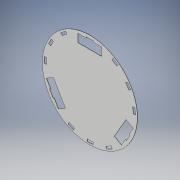
# Autodesk Inventor part: Part2
Saved by Autodesk Inventor 2019 (Build 230136000, 136)
## iProperties
Created: 2021-01-08
Part Number: Part2
Material: Generic
Document SubType Name: Modeling
Designer: DELL
Density: 1 g/cm^3
Appearance: Default
Author: DELL
Autodesk Inventor part; units mm, degrees
ref_plane "YZ Plane" through (0, 0, 0) normal (1, 0, 0) x (0, 1, 0)
ref_plane "XZ Plane" through (0, 0, 0) normal (0, 1, 0) x (-1, 0, 0)
ref_plane "XY Plane" through (0, 0, 0) normal (0, 0, 1) x (1, 0, 0)
sketch "Sketch1" plane through (0, 0, 0) normal (0, 0, 1) x (1, 0, 0)
  circle A0 centre (0, 0) radius 200
  line L0 (0, 187.7709) -> (15, 187.7709)
  line L1 (15, 187.7709) -> (15, 182.7709)
  line L2 (15, 182.7709) -> (50, 182.7709)
  line L3 (50, 182.7709) -> (50, 147.7709)
  line L4 (50, 147.7709) -> (-50, 147.7709)
  line L5 (-50, 147.7709) -> (-50, 182.7709)
  line L6 (-50, 182.7709) -> (-15, 182.7709)
  line L7 (-15, 182.7709) -> (-15, 187.7709)
  line L8 (-15, 187.7709) -> (0, 187.7709)
  line L9 (-162.6144, -93.8855) -> (-170.1144, -80.8951)
  line L10 (-170.1144, -80.8951) -> (-165.7843, -78.3951)
  line L11 (-165.7843, -78.3951) -> (-183.2843, -48.0842)
  line L12 (-183.2843, -48.0842) -> (-152.9734, -30.5842)
  line L13 (-152.9734, -30.5842) -> (-102.9734, -117.1867)
  line L14 (-102.9734, -117.1867) -> (-133.2843, -134.6867)
  line L15 (-133.2843, -134.6867) -> (-150.7843, -104.3758)
  line L16 (-150.7843, -104.3758) -> (-155.1144, -106.8758)
  line L17 (-155.1144, -106.8758) -> (-162.6144, -93.8855)
  line L18 (162.6144, -93.8855) -> (155.1144, -106.8758)
  line L19 (155.1144, -106.8758) -> (150.7843, -104.3758)
  line L20 (150.7843, -104.3758) -> (133.2843, -134.6867)
  line L21 (133.2843, -134.6867) -> (102.9734, -117.1867)
  line L22 (102.9734, -117.1867) -> (152.9734, -30.5842)
  line L23 (152.9734, -30.5842) -> (183.2843, -48.0842)
  line L24 (183.2843, -48.0842) -> (165.7843, -78.3951)
  line L25 (165.7843, -78.3951) -> (170.1144, -80.8951)
  line L26 (170.1144, -80.8951) -> (162.6144, -93.8855)
  line L27 (12.5, 183.7364) -> (12.5, 193.7364)
  line L28 (-173.6251, 83.379) -> (-162.3777, 105.706)
  line L29 (-162.3777, 105.706) -> (-153.4469, 101.2071)
  line L30 (-153.4469, 101.2071) -> (-164.6943, 78.88)
  line L31 (-164.6943, 78.88) -> (-173.6251, 83.379)
  line L32 (-181.8421, 26.8753) -> (-182.5998, 1.8868)
  line L33 (-192.5952, 2.1899) -> (-191.8375, 27.1784)
  line L34 (-182.5998, 1.8868) -> (-192.5952, 2.1899)
  line L35 (-191.8375, 27.1784) -> (-181.8421, 26.8753)
  line L36 (-115.9276, 141.0924) -> (-122.1203, 148.9442)
  line L37 (-96.2982, 156.5742) -> (-115.9276, 141.0924)
  line L38 (-102.4909, 164.426) -> (-96.2982, 156.5742)
  line L39 (-122.1203, 148.9442) -> (-102.4909, 164.426)
  line L40 (72.3815, -179.7253) -> (67.6463, -170.9175)
  line L41 (67.6463, -170.9175) -> (89.6659, -159.0795)
  line L42 (94.4011, -167.8873) -> (72.3815, -179.7253)
  line L43 (89.6659, -159.0795) -> (94.4011, -167.8873)
  line L44 (14.035, -182.0694) -> (14.6042, -192.0532)
  line L45 (-10.9244, -183.4924) -> (14.035, -182.0694)
  line L46 (-10.3552, -193.4762) -> (-10.9244, -183.4924)
  line L47 (14.6042, -192.0532) -> (-10.3552, -193.4762)
  line L48 (-64.2258, -170.9424) -> (-67.9293, -180.2313)
  line L49 (-87.4482, -161.6838) -> (-64.2258, -170.9424)
  line L50 (-67.9293, -180.2313) -> (-91.1516, -170.9727)
  line L51 (-91.1516, -170.9727) -> (-87.4482, -161.6838)
  line L52 (119.4559, 152.5469) -> (114.1957, 144.0422)
  line L53 (114.1957, 144.0422) -> (92.9339, 157.1927)
  line L54 (98.1941, 165.6974) -> (119.4559, 152.5469)
  line L55 (92.9339, 157.1927) -> (98.1941, 165.6974)
  line L56 (150.6592, 103.1894) -> (159.0209, 108.6742)
  line L57 (164.3713, 82.2854) -> (150.6592, 103.1894)
  line L58 (172.7329, 87.7702) -> (164.3713, 82.2854)
  line L59 (159.0209, 108.6742) -> (172.7329, 87.7702)
  line L60 (180.1534, 29.85) -> (190.0496, 31.2872)
  line L61 (183.7463, 5.1095) -> (180.1534, 29.85)
  line L62 (190.0496, 31.2872) -> (193.6425, 6.5467)
  line L63 (193.6425, 6.5467) -> (183.7463, 5.1095)
  point P0 (-163.536, 92.293)
  point P1 (-187.2187, 14.5326)
  point P2 (-109.2092, 152.7592)
  point P3 (81.0237, -169.4024)
  point P4 (1.8399, -187.7728)
  point P5 (-77.6887, -170.9575)
  point P6 (106.1949, 154.8698)
  point P7 (161.6961, 95.4798)
  point P8 (186.8979, 18.1984)
  dimension "d12" = 360
  dimension "d28" = 25
  dimension "d32" = 25
  dimension "d36" = 360
  constraints: 128 end point, 8 perpendicular, 6 coincident, 3 point on line, 2 parallel, 1 centre point, 1 horizontal, 161 other
extrude "Extrusion1" add sketch "Sketch1" along normal blind 1.5
body "Solid1"
